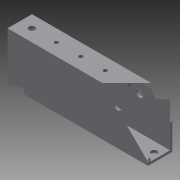
# Autodesk Inventor part: frame_front_bumper
Saved by Autodesk Inventor 2015 SP1 (Build 190203100, 203)
## iProperties
Created: 2014-12-23
Part Number: frame_front_bumper
Material: Generic
Document SubType Name: Modeling
Designer: Jarod
Density: 1 g/cm^3
Appearance: Default
Author: Jarod
Autodesk Inventor part; units mm, degrees
ref_plane "YZ Plane" through (0, 0, 0) normal (1, 0, 0) x (0, 1, 0)
ref_plane "XZ Plane" through (0, 0, 0) normal (0, 1, 0) x (-1, 0, 0)
ref_plane "XY Plane" through (0, 0, 0) normal (0, 0, 1) x (1, 0, 0)
sketch "Sketch1" plane through (0, 0, 0) normal (1, 0, 0) x (0, 1, 0)
  line L0 (0, 0) -> (50.8, 0)
  line L1 (50.8, 0) -> (50.8, -25.4)
  line L2 (50.8, -25.4) -> (0, -25.4)
  line L3 (0, -25.4) -> (0, 0)
  line L4 (2.54, -2.54) -> (48.26, -2.54)
  line L5 (48.26, -2.54) -> (48.26, -22.86)
  line L6 (48.26, -22.86) -> (2.54, -22.86)
  line L7 (2.54, -22.86) -> (2.54, -2.54)
  dimension "d0" = 50.8
  dimension "d1" = 25.4
  dimension "d2" = 45.72
  dimension "d3" = 20.32
  dimension "d4" = 2.54
  dimension "d5" = 2.54
  constraints: 16 end point, 4 parallel, 2 horizontal, 2 perpendicular
  measures "d0" distance of L1.end L2.end
  measures "d1" distance of L0.end L1.end
  measures "d2" distance of L5.end L6.end
  measures "d3" distance of L4.end L5.end
  measures "d4" distance between parallel lines of L7 L3
  measures "d5" distance between parallel lines of L0 L4
extrude "Extrusion1" add sketch "Sketch1" along normal blind 146.05
sketch "Sketch5" plane through (0, 50.8, 0) normal (0, 1, 0) x (1, 0, 0)
  line L0 (0, 0) -> (0, 25.4) projected
  line L1 (0, 0) -> (146.05, 0) projected
  line L2 (146.05, 25.4) -> (146.05, 0) projected
  line L3 (0, 25.4) -> (146.05, 25.4) projected
  point P0 (12.7, 12.7)
  dimension "d39" = 12.7
  dimension "d40" = 12.7
  measures "d39" distance from line of L3 point (12.7, 12.7)
  measures "d40" distance from line of L0 point (12.7, 12.7)
hole "Hole3" at (12.7, 50.8, -12.7) direction (0, -1, 0) diameter 3.9688 end through all
pattern_linear "Rectangular Pattern1" count 6 spacing 25.4 along (1, 0, 0) of "Hole3"
sketch "Sketch6" plane through (0, 0, -25.4) normal (0, 0, -1) x (-1, 0, 0)
  line L0 (0, 50.8) -> (0, 0) projected
  line L1 (0, 50.8) -> (-146.05, 50.8) projected
  line L2 (-146.05, 0) -> (-146.05, 50.8) projected
  line L3 (0, 0) -> (-146.05, 0) projected
  point P0 (-114.3, 38.1)
  dimension "d51" = 12.7
  dimension "d52" = 31.75
  measures "d51" distance from line of L1 point (-114.3, 38.1)
  measures "d52" distance from line of point (-114.3, 38.1) L2
hole "Hole4" at (114.3, 38.1, -25.4) direction (0, 0, 1) diameter 7.9375 end through all
sketch "Sketch7" plane through (0, 50.8, 0) normal (0, 1, 0) x (1, 0, 0)
  circle A0 centre (139.7, 12.7) radius 1.9844 projected
  circle A1 centre (114.3, 12.7) radius 1.9844 projected
  circle A2 centre (88.9, 12.7) radius 1.9844 projected
  circle A3 centre (63.5, 12.7) radius 1.9844 projected
  circle A4 centre (38.1, 12.7) radius 1.9844 projected
  circle A5 centre (12.7, 12.7) radius 1.9844 projected
  line L0 (0, 0) -> (0, 25.4) projected
  line L1 (0, 0) -> (146.05, 0) projected
  line L2 (146.05, 25.4) -> (146.05, 0) projected
  line L3 (0, 25.4) -> (146.05, 25.4) projected
  circle A6 centre (12.7, 12.7) radius 1.9844 projected
  circle A7 centre (12.7, 12.7) radius 3.175
  circle A8 centre (139.7, 12.7) radius 3.175
  dimension "d60" = 6.35
  dimension "d61" = 6.35
  constraints: 2 centre point, 2 coincident
  measures "d60" diameter of A7
  measures "d61" diameter of A8
extrude "Extrusion3" cut sketch "Sketch7" against normal blind 50.8 contours A7 | A8
sketch "Sketch8" plane through (0, 0, -25.4) normal (0, 0, -1) x (-1, 0, 0)
  circle A0 centre (-114.3, 38.1) radius 3.9687 projected
  line L0 (0, 50.8) -> (0, 0) projected
  line L1 (0, 50.8) -> (-146.05, 50.8) projected
  line L2 (-146.05, 0) -> (-146.05, 50.8) projected
  line L3 (0, 0) -> (-146.05, 0) projected
  point P0 (-25.4, 31.75)
  dimension "d64" = 19.05
  dimension "d65" = 25.4
  measures "d64" distance from line of point (-25.4, 31.75) L1
  measures "d65" distance from line of L0 point (-25.4, 31.75)
hole "Hole5" at (25.4, 31.75, -25.4) direction (0, 0, 1) diameter 7.9375 end through all
body "Solid1"
